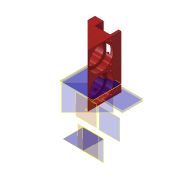
# Autodesk Inventor part: 30_Cube_Insert_Filter_Revolver_Filter_base_triple
Saved by Autodesk Inventor 2022 (Build 260153000, 153)
## iProperties
Created: 2021-09-13
Part Number: 30_Cube_Insert_Filter_Revolver_Filter_base_triple
Material: Generic
Document SubType Name: Modeling
Designer: diederichbenedict
Density: 1 g/cm^3
Appearance: Rot
Mass: 6.97028 g
Surface Area: 48.8121 cm^2
Volume: 6.97028 cm^3
Author: diederichbenedict
Autodesk Inventor part; units mm, degrees
ref_plane "YZ Plane" through (0, 0, 0) normal (1, 0, 0) x (0, 1, 0)
ref_plane "XZ Plane" through (0, 0, 0) normal (0, 1, 0) x (-1, 0, 0)
ref_plane "XY Plane" through (0, 0, 0) normal (0, 0, 1) x (1, 0, 0)
ref_plane "Work Plane1" through (-34.3358, -34.38, 2.0699) normal (0, -1, 0) x (0.7071068, 0, -0.7071068)
ref_plane "Work Plane4" through (-9.5871, -34.38, 28.2329) normal (0, -1, 0) x (1, 0, 0)
ref_plane "Work Plane3" through (-9.5871, -32.38, 28.2329) normal (0, -1, 0) x (1, 0, 0)
sketch "Sketch1" plane through (-9.5871, -34.38, 28.2329) normal (0, -1, 0) x (1, 0, 0)
  line L0 (0.7071, -1.3185) -> (0.7071, -26.3185) construction
  line L1 (0.7071, -1.3185) -> (1.7071, -1.3185) construction
  line L2 (0.7071, -26.3185) -> (1.7071, -26.3185) construction
  line L3 (-4.2929, -0.7071) -> (-31.7929, -28.2071)
  line L4 (-31.7929, -28.2071) -> (0.7071, -28.2071)
  line L5 (0.7071, -28.2071) -> (0.7071, -0.7071)
  line L6 (0.7071, -0.7071) -> (-4.2929, -0.7071)
  line L7 (-4.2929, -0.7071) -> (-4.2929, -28.2071)
  line L8 (-4.2929, -28.2071) -> (0.7071, -28.2071)
  line L9 (0.7071, -0.7071) -> (3.5978, -0.7071)
  line L10 (2.5336, 1.8671) -> (2.3871, 1.8671) projected
  line L11 (0.7071, -0.7071) -> (0.7071, -28.2071)
  line L12 (0.7071, -28.2071) -> (-31.7929, -28.2071)
  point P0 (9.5871, -28.2329)
  dimension "d1" = 5
  dimension "d96" = 27.5
  dimension "d97" = 135
  constraints: 22 end point, 4 perpendicular, 3 horizontal, 2 point on line, 1 collinear, 2 other
  measures "d1" distance of L5.end L3.start
  measures "d96" distance between parallel lines of L4 L6
  measures "d97" angle of L7 L3
extrude "Extrusion1" add sketch "Sketch1" against normal blind 28
ref_plane "Work Plane5" through (-9.5871, -20.38, 28.2329) normal (0, -1, 0) x (1, 0, 0)
ref_plane "Work Plane6" through (-11.0013, -34.38, 27.5258) normal (0, 0, 1) x (1, 0, 0)
sketch "Sketch4" plane through (-8.88, -34.38, 27.5258) normal (-1, 0, 0) x (0, 0, 1)
  circle A0 centre (-13.75, 14) radius 10
  line L0 (0, 0) -> (0, 28) projected
  point P0 (-27.5258, 34.38)
  dimension "d90" = 20
  dimension "d98" = 13.75
  constraints: 1 centre point
  measures "d90" diameter of A0
  measures "d98" distance from line of A0.centre L0
extrude "Extrusion4" cut sketch "Sketch4" along normal through all
sketch "Sketch9" plane through (-11.38, -34.38, 30.0258) normal (-0.7071068, 0, 0.7071068) x (0.7071068, 0, 0.7071068)
  ellipse E0 centre (-22.981, 14) end of major axis (-37.1231, 14) minor radius 10 projected
  line L0 (-3.5355, 0) -> (-42.4264, 0) projected
  line L1 (-3.5355, 0) -> (-3.5355, 28) projected
  line L2 (-42.4264, 28) -> (-3.5355, 28) projected
  line L3 (-42.4264, 0) -> (-42.4264, 28) projected
  line L4 (0, 0) -> (-3.5355, 0) projected
  line L5 (0, 0) -> (0, 28) projected
  line L6 (-3.5355, 28) -> (0, 28) projected
  line L7 (-3.5355, 0) -> (-3.5355, 28) projected
  point P0 (-13.1846, 34.38)
  point P1 (-3.5355, 0)
  constraints: 1 other
extrude "Extrusion9" cut sketch "Sketch9" against normal blind 3.3 contours E0 | L0 L3 L2 L1 | L1 L6 L5 L4
sketch "Sketch3" plane through (-8.88, -34.38, 27.5258) normal (-1, 0, 0) x (0, 0, 1)
  circle A0 centre (-13.75, 14) radius 10 projected
  circle A1 centre (-13.75, 14) radius 13
  circle A2 centre (-23.75, 3) radius 1.4
  circle A3 centre (-23.75, 25) radius 1.4
  line L0 (22.7337, 14) -> (-44.6223, 14) projected
  point P0 (-27.5258, 34.38)
  point P1 (13.1114, 14)
  dimension "d100" = 26
  dimension "d178" = 2.8
  dimension "d179" = 2.8
  dimension "d180" = 11
  dimension "d181" = 11
  dimension "d182" = 10
  dimension "d183" = 10
  constraints: 3 centre point, 1 coincident
  measures "d100" diameter of A1
  measures "d178" diameter of A2
  measures "d179" diameter of A3
  measures "d180" distance from line of A2.centre L0
  measures "d181" distance from line of A3.centre L0
  measures "d182" horizontal distance of A3.centre A0.centre
  measures "d183" horizontal distance of A0.centre A2.centre
extrude "Extrusion3" cut sketch "Sketch3" along normal blind 7
sketch "Sketch13" plane through (-10.0465, -34.38, 26.6923) normal (-0.7071068, 0, 0.7071068) x (0.7071068, 0, 0.7071068)
  line L0 (-8.2497, 3.0991) -> (-8.2497, 6.941) projected
  ellipse E0 centre (-18.2668, 14) end of major axis (-32.4089, 14) minor radius 10 (-8.2497, 21.059) -> (-8.2497, 6.941) ccw projected
  line L1 (-8.2497, 21.059) -> (-8.2497, 24.9009) projected
  ellipse E1 centre (-18.2668, 14) end of major axis (0.118, 14) minor radius 13 (-8.2497, 3.0991) -> (-8.2497, 24.9009) ccw projected
  line L2 (-37.7122, 0) -> (-37.7122, 28) projected
  line L3 (1.1787, 0) -> (-37.7122, 0) projected
  line L4 (1.1787, 28) -> (1.1787, 0) projected
  line L5 (-37.7122, 28) -> (1.1787, 28) projected
  circle A0 centre (-32.7122, 25.5) radius 1.4
  circle A1 centre (-32.7122, 2.5) radius 1.4
  line L6 (9.2395, 0) -> (-45.5375, 0) projected
  dimension "d142" = 2.8
  dimension "d143" = 2.8
  dimension "d144" = 2.5
  dimension "d146" = 5
  dimension "d147" = 2.5
  dimension "d148" = 5
  constraints: 2 centre point, 2 other
  measures "d142" diameter of A0
  measures "d143" diameter of A1
  measures "d144" distance from line of A0.centre L5
  measures "d146" distance from line of L2 A0.centre
  measures "d147" distance from line of L6 A1.centre
  measures "d148" distance from line of L2 A1.centre
extrude "Extrusion13" cut sketch "Sketch13" against normal blind 10 contours A0 | A1
ref_plane "Arbeitsebene13" through (-3.6065, -62.7242, 27.5258) normal (0, 0, -1) x (-1, 0, 0)
ref_plane "Arbeitsebene16" through (-8.88, -62.38, 27.5258) normal (0, 0, 1) x (1, 0, 0)
ref_plane "Work Plane11" through (-8.88, -20.38, 27.5258) normal (0, -1, 0) x (1, 0, 0)
ref_plane "Arbeitsebene12" through (-8.88, -20.38, 27.5258) normal (0, -1, 0) x (1, 0, 0)
ref_plane "Arbeitsebene15" through (-13.88, -62.38, 0.0258) normal (0, 0, -1) x (1, 0, 0)
sketch "Skizze20" plane through (-13.88, -62.38, 0.0258) normal (0, 0, -1) x (1, 0, 0)
  circle A0 centre (27.7649, 33.0797) radius 1.45
  point P0 (13.88, -62.38)
  dimension "d93" = 2.9
  constraints: 1 centre point
  measures "d93" diameter of A0
extrude "Extrusion17" cut sketch "Skizze20" against normal blind 10
ref_plane "Arbeitsebene14" through (-13.88, -62.38, 27.5258) normal (0, -1, 0) x (1, 0, 0)
ref_plane "Arbeitsebene17" through (-13.88, -62.38, 27.5258) normal (0, -1, 0) x (1, 0, 0)
sketch "Skizze25" plane through (-9.5871, -34.38, 28.2329) normal (0, -1, 0) x (1, 0, 0)
  line L0 (0.374, -0.7071) -> (-27.126, -28.2071) projected
  line L1 (-27.126, -28.2071) -> (0.7071, -28.2071) projected
  line L2 (0.7071, -28.2071) -> (0.7071, -0.7071) projected
  line L3 (0.7071, -0.7071) -> (0.374, -0.7071) projected
  line L4 (-2.0328, -29.7071) -> (-18.0328, -29.7071)
  line L5 (-18.0328, -29.7071) -> (-18.0328, -26.7071)
  line L6 (-18.0328, -26.7071) -> (-2.0328, -26.7071)
  line L7 (-2.0328, -26.7071) -> (-2.0328, -29.7071)
  line L8 (0.7071, -28.2071) -> (-27.126, -28.2071) projected
  line L9 (-2.0328, -29.7071) -> (-18.0328, -26.7071) construction
  line L10 (-18.0328, -29.7071) -> (-2.0328, -26.7071) construction
  point P0 (9.5871, -28.2329)
  point P1 (-10.0328, -28.2071)
  dimension "d149" = 16
  dimension "d150" = 3
  constraints: 12 end point, 2 midpoint, 2 parallel, 1 horizontal, 1 perpendicular, 1 point on line
  measures "d149" distance of L5.end L6.end
  measures "d150" distance of L4.end L5.end
extrude "Extrusion21" cut sketch "Skizze25" against normal through all contours L5 L6 L7 L1 | L1 L7 L4 L5
pattern_linear "Rechteckige Anordnung5" count 2 spacing 28 along (0, 1, 0) of "Extrusion21", "Extrusion17", "Extrusion13", "Extrusion9", "Extrusion1", "Extrusion3", "Extrusion4"
sketch "Skizze26" plane through (-9.5871, -34.38, 28.2329) normal (0, -1, 0) x (1, 0, 0)
  circle A0 centre (-10.1167, -19.4776) radius 1.635
  point P0 (9.5871, -28.2329)
  constraints: 1 centre point
extrude "Extrusion22" cut sketch "Skizze26" against normal blind 10 draft -2
sketch "Skizze27" plane through (-9.5871, -34.38, 28.2329) normal (0, -1, 0) x (1, 0, 0)
  line L0 (-11.8828, -27.7371) -> (-8.2828, -27.7371) projected
  line L1 (-8.2828, -27.7371) -> (-8.2828, -23.5571) projected
  line L2 (-8.2828, -23.5571) -> (-0.6428, -23.5571) projected
  line L3 (-0.6428, -23.5571) -> (-0.6428, -15.7571) projected
  line L4 (-0.6428, -15.7571) -> (-19.5228, -15.7571) projected
  line L5 (-19.5228, -15.7571) -> (-19.5228, -23.5571) projected
  line L6 (-19.5228, -23.5571) -> (-11.8828, -23.5571) projected
  line L7 (-11.8828, -23.5571) -> (-11.8828, -27.7371) projected
  line L8 (-2.7178, -27.7371) -> (-17.4478, -27.7371) projected
  line L9 (-17.4478, -27.7371) -> (-17.4478, -38.5671) projected
  line L10 (-17.4478, -38.5671) -> (-2.7178, -38.5671) projected
  line L11 (-2.7178, -38.5671) -> (-2.7178, -27.7371) projected
  circle A0 centre (-10.0828, -31.2171) radius 1.5 projected
  circle A1 centre (-14.9928, -34.9671) radius 1.25 construction
  circle A2 centre (-5.1728, -34.9671) radius 1.25 construction
  circle A3 centre (-10.1167, -19.4776) radius 1.635 projected
  line L12 (-18.0328, -28.2071) -> (-18.0328, -26.7071) projected
  line L13 (-18.0328, -26.7071) -> (-2.0328, -26.7071) projected
  line L14 (-2.0328, -26.7071) -> (-2.0328, -28.2071) projected
  line L15 (-2.0328, -28.2071) -> (0.7071, -28.2071) projected
  line L16 (0.7071, -28.2071) -> (0.7071, -0.7071) projected
  line L17 (0.7071, -0.7071) -> (0.374, -0.7071) projected
  line L18 (0.374, -0.7071) -> (-27.126, -28.2071) projected
  line L19 (-27.126, -28.2071) -> (-18.0328, -28.2071) projected
  line L20 (-27.126, -28.2071) -> (-18.0328, -28.2071) projected
  line L21 (-27.126, -28.2071) -> (-17.4478, -28.2071)
  line L22 (-17.4478, -28.2071) -> (-17.4478, -35.7071)
  line L23 (-17.4478, -35.7071) -> (-27.126, -35.7071)
  line L24 (-27.126, -35.7071) -> (-27.126, -28.2071)
  line L25 (0.7071, -28.2071) -> (-2.7178, -28.2071)
  line L26 (-2.7178, -28.2071) -> (-2.7178, -35.7071)
  line L27 (-2.7178, -35.7071) -> (0.7071, -35.7071)
  line L28 (0.7071, -35.7071) -> (0.7071, -28.2071)
  line L29 (-17.4478, -35.7071) -> (-16.0002, -35.7071)
  line L30 (-13.9854, -35.7071) -> (-6.1802, -35.7071)
  line L31 (-4.1654, -35.7071) -> (-2.7178, -35.7071)
  circle A4 centre (-10.0828, -31.2171) radius 2.1
  line L32 (-12.1828, -38.5671) -> (-12.1828, -31.2171)
  line L33 (-7.9828, -31.2171) -> (-7.9828, -38.5671)
  circle A5 centre (-14.9928, -34.9671) radius 1.75
  circle A6 centre (-5.1728, -34.9671) radius 1.75
  point P0 (9.5871, -28.2329)
  point P1 (-12.1828, -35.7071)
  point P2 (-7.9828, -35.7071)
  point P3 (-16.5787, -35.7071)
  point P4 (-13.407, -35.7071)
  point P5 (-6.7587, -35.7071)
  point P6 (-3.587, -35.7071)
  point P7 (-2.7178, -28.2071)
  dimension "d159" = 7.5
  dimension "d163" = 0.6
  dimension "d164" = 3.5
  dimension "d165" = 3.5
  constraints: 26 end point, 12 point on line, 10 point on circle, 4 parallel, 3 centre point, 3 horizontal, 3 perpendicular, 2 coincident, 1 collinear, 1 tangent
  measures "d159" distance of L21.end L22.end
  measures "d163" radial gap between concentric circles of A0 A4
  measures "d164" diameter of A5
  measures "d165" diameter of A6
extrude "Extrusion23" add sketch "Skizze27" against normal blind 30 contours L7 L13 L1 L0 | L8 L9 L21 L12 L13 L7 | L0 L8 L11 L31 A6 L30 L33 A4 L32 A5 L29 L9 | L1 L13 L14 L25 L11 L8 | L9 L23 L24 L19 L21 | L25 L15 L28 L27 L11
sketch "Skizze28" plane through (-9.5871, -4.38, 28.2329) normal (0, 1, 0) x (1, 0, 0)
  circle A0 centre (-14.9928, 34.9671) radius 1.55 projected
  circle A1 centre (-5.1728, 34.9671) radius 1.55 projected
  circle A2 centre (-10.0828, 31.2171) radius 1.5 projected
  line L0 (-2.5328, 41.7171) -> (-17.6328, 41.7171) projected
  line L1 (-17.6328, 41.7171) -> (-17.6328, 27.2071) projected
  line L2 (-17.6328, 27.2071) -> (-2.5328, 27.2071) projected
  line L3 (-2.5328, 41.7171) -> (-2.5328, 27.2071) projected
  line L4 (0.7071, 28.2071) -> (-2.0328, 28.2071) projected
  line L5 (0.7071, 28.2071) -> (0.7071, 35.7071) projected
  line L6 (0.7071, 35.7071) -> (-3.587, 35.7071) projected
  arc A3 (-6.7587, 35.7071) -> (-3.587, 35.7071) centre (-5.1728, 34.9671) ccw projected
  line L7 (-6.7587, 35.7071) -> (-7.9828, 35.7071) projected
  line L8 (-7.9828, 35.7071) -> (-7.9828, 31.2171) projected
  arc A4 (-12.1828, 31.2171) -> (-7.9828, 31.2171) centre (-10.0828, 31.2171) ccw projected
  line L9 (-12.1828, 31.2171) -> (-12.1828, 35.7071) projected
  line L10 (-12.1828, 35.7071) -> (-13.407, 35.7071) projected
  arc A5 (-16.5787, 35.7071) -> (-13.407, 35.7071) centre (-14.9928, 34.9671) ccw projected
  line L11 (-16.5787, 35.7071) -> (-27.126, 35.7071) projected
  line L12 (-27.126, 35.7071) -> (-27.126, 28.2071) projected
  line L13 (-21.9042, 28.2071) -> (-27.126, 28.2071) projected
  line L14 (-21.9042, 28.2071) -> (-18.2056, 28.2071) projected
  line L15 (-18.0328, 28.2071) -> (-18.2056, 28.2071) projected
  line L16 (-18.0328, 26.7071) -> (-18.0328, 28.2071) projected
  line L17 (-2.0328, 26.7071) -> (-18.0328, 26.7071) projected
  line L18 (-2.0328, 28.2071) -> (-2.0328, 26.7071) projected
  line L19 (-21.9042, 28.2071) -> (-27.126, 28.2071) projected
  line L20 (-27.126, 28.2071) -> (-18.0328, 28.2071)
  line L21 (-18.0328, 28.2071) -> (-18.0328, 35.7071)
  line L22 (-18.0328, 35.7071) -> (-27.126, 35.7071)
  line L23 (-27.126, 35.7071) -> (-27.126, 28.2071)
  line L24 (0.7071, 28.2071) -> (-2.0328, 28.2071) projected
  line L25 (-3.587, 35.7071) -> (0.7071, 35.7071) projected
  line L26 (-2.0328, 28.2071) -> (0.7071, 28.2071)
  line L27 (0.7071, 28.2071) -> (0.7071, 35.7071)
  line L28 (0.7071, 35.7071) -> (-2.0328, 35.7071)
  line L29 (-2.0328, 35.7071) -> (-2.0328, 28.2071)
  point P0 (9.5871, 28.2329)
  point P1 (-2.0328, 35.7071)
  constraints: 16 end point, 4 parallel, 2 horizontal, 2 perpendicular, 1 point on line
extrude "Extrusion24" add sketch "Skizze28" along normal up to surface (26 mm away) contours L6 L5 L4 L29 | L21 L15 L14 L13 L12 L11
sketch "Skizze29" plane through (-8.88, -34.38, 27.5258) normal (1, 0, 0) x (0, 0, -1)
  circle A0 centre (13.75, 14) radius 13 projected
  point P0 (27.5258, 34.38)
extrude "Extrusion25" cut sketch "Skizze29" against normal up to surface (7 mm away)
sketch "Skizze30" plane through (-26.1658, -34.38, -7.4742) normal (0, 0, -1) x (-1, 0, 0)
  line L0 (10.5473, 0) -> (0, 0) projected
  line L1 (10.5473, 0) -> (10.5473, 56) projected
  line L2 (10.5473, 56) -> (1.4542, 56) projected
  line L3 (1.4542, 30) -> (1.4542, 56) projected
  line L4 (0, 30) -> (1.4542, 30) projected
  line L5 (0, 0) -> (0, 30) projected
  ellipse E0 centre (3.4763, 25.5) end of major axis (1.4964, 25.5) minor radius 1.4 projected
  circle A0 centre (1.5257, 25.2601) radius 1.4
  circle A1 centre (1.6781, 5.3947) radius 1.4
  circle A2 centre (1.6781, 14.2382) radius 1.4
  circle A3 centre (-14.3297, 25.2601) radius 1.4
  circle A4 centre (-14.1784, 14.2382) radius 1.4
  circle A5 centre (-14.1784, 5.3947) radius 1.4
  point P0 (-26.1658, 34.38)
  dimension "d170" = 2.8
  dimension "d171" = 2.8
  dimension "d174" = 2.8
  dimension "d175" = 2.8
  dimension "d176" = 2.8
  dimension "d177" = 2.8
  constraints: 6 centre point, 2 other
  measures "d170" diameter of A0
  measures "d171" diameter of A1
  measures "d174" diameter of A2
  measures "d175" diameter of A3
  measures "d176" diameter of A4
  measures "d177" diameter of A5
extrude "Extrusion26" cut sketch "Skizze30" against normal blind 6 contours E0 A0 | E0 A0 | A1 | A2 | A3 | A4 | A5 picked at (2.3908, 25.6477) picked at (0.6011, 25.21)
ref_plane "Work Plane2" through (41.82, -7.88, -4) normal (0, -1, 0) x (1, 0, 0)
equation "\"d98\" = 0.5 * d96"
equation "\"d147\" = d144"
equation "\"d148\" = d146"
body "Solid1"
